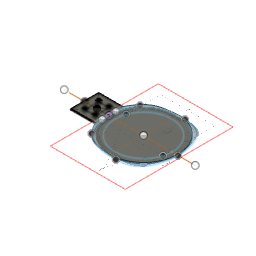
Support Joystick v4 (Autodesk Fusion 360 design; units mm, degrees)
Autodesk Fusion 360 part; units mm, degrees
sketch "Esquisse2" plane through (0, 0, 0) normal (0, 0, 1) x (1, 0, 0)
  line L0 (0, 0) -> (-70, 0)
  circle A0 centre (100, 0) radius 82.5
  line L1 (250, 0) -> (-130, 0)
  spline S0 degree 5 poles (0, 20) (0, 22.4882) (0.1779, 27.4114) (0.975, 34.6277) (3.4457, 44.3914) (10.1068, 57.8847) (21.3924, 73.1358) (35.9935, 85.4932) (52.8737, 92.6951) (72.095, 96.3693) (93.5882, 98.471) (117.0022, 100.5708) (140.5192, 100.2508) (161.4884, 92.9068) (178.6566, 78.1832) (191.1793, 56.7401) (197.2314, 35.6259) (199.4965, 18.2943) (200, 6.1899) (200, 0) knots 0 0 0 0 0 0 0.066667 0.133333 0.2 0.266667 0.333333 0.4 0.466667 0.533333 0.6 0.666667 0.733333 0.8 0.866667 0.933333 1 1 1 1 1 1
  line L2 (0, 0) -> (0, 40)
  line L3 (96.4605, 99.786) -> (143.5395, 100.214)
  line L4 (4.3857, 52.2523) -> (35.6143, 87.7477)
  spline S1 degree 5 poles (0, -20) (0, -22.4882) (0.1779, -27.4114) (0.975, -34.6277) (3.4457, -44.3914) (10.1068, -57.8847) (21.3924, -73.1358) (35.9935, -85.4932) (52.8737, -92.6951) (72.095, -96.3693) (93.5882, -98.471) (117.0022, -100.5708) (140.5192, -100.2508) (161.4884, -92.9068) (178.6566, -78.1832) (191.1793, -56.7401) (197.2314, -35.6259) (199.4965, -18.2943) (200, -6.1899) (200, 0) knots 0 0 0 0 0 0 0.066667 0.133333 0.2 0.266667 0.333333 0.4 0.466667 0.533333 0.6 0.666667 0.733333 0.8 0.866667 0.933333 1 1 1 1 1 1
  line L5 (200, 30) -> (200, -30)
  line L6 (0, 0) -> (0, -40)
  line L7 (4.3857, -52.2523) -> (35.6143, -87.7477)
  line L8 (96.4605, -99.786) -> (143.5395, -100.214)
  line L9 (200, -30) -> (200, 30)
  circle A1 centre (22.2756, 27.6617) radius 3.1
  circle A2 centre (179.3345, -22.6338) radius 3.1
  ellipse E0 centre (100, 0) end of major axis (100, 100) minor radius 100
  line L10 (100, -100) -> (100, 100)
  line L11 (200, 0) -> (0, 0)
  line L12 (-70, 40) -> (0, 40)
  line L13 (0, 40) -> (0, -40)
  line L14 (0, -40) -> (-70, -40)
  line L15 (-70, -40) -> (-70, 40)
  line L16 (-70, 40) -> (0, -40) construction
  line L17 (0, 40) -> (-70, -40) construction
  line L18 (0, -40) -> (10.9445, -57.8049)
  line L19 (0, 40) -> (10.9445, 57.8049)
  line L20 (-20, -20) -> (-50, -20)
  line L21 (-50, -20) -> (-50, 20)
  line L22 (-50, 20) -> (-20, 20)
  line L23 (-20, 20) -> (-20, -20)
  circle A3 centre (-50, 20) radius 4
  circle A4 centre (-20, 20) radius 4
  circle A5 centre (-50, -20) radius 4
  circle A6 centre (-20, -20) radius 4
  point P0 (-35, 0)
  point P1 (20, 70)
  point P2 (120, 100)
  point P3 (20, -70)
  point P4 (120, -100)
  point P5 (-35, 0)
  dimension "d3" = 70
  dimension "d5" = 165
  dimension "d6" = 6.2
  dimension "d7" = 6.2
  dimension "d18" = 70
  dimension "d19" = 80
  dimension "d28" = 20
  dimension "d29" = 8
  dimension "d32" = 30
  dimension "d33" = -40
  constraint coincident L0.start L2.start
  constraint horizontal L0
  constraint midpoint L0 P5
  constraint coincident L1 S0.end
  constraint midpoint S0.start L2
  constraint perpendicular L0 L2
  constraint midpoint P2 L3
  constraint midpoint P1 L4
  constraint midpoint S0.end L5
  constraint symmetric S0.start L1 S1.start
  constraint symmetric L1 P1 P3
  constraint symmetric L1 P2 P4
  constraint symmetric L1 L0.start L2.start
  constraint symmetric L1 L2.end L6.end
  constraint symmetric L1 L3.start L8.start
  constraint symmetric L1 L3.end L8.end
  constraint symmetric L1 L4.start L7.start
  constraint symmetric L1 L4.end L7.end
  constraint symmetric L1 L5.start L5.end
  constraint symmetric L1 L5.end L5.start
  constraint coincident A0 A1.centre
  constraint coincident A0 A2.centre
  constraint coincident E0 L10.start
  constraint coincident E0 L10.end
  constraint coincident S0.end E0
  constraint coincident L0.start E0
  constraint concentric A0 E0
  constraint perpendicular L1 L10
  constraint horizontal L12
  constraint perpendicular L12 L13
  constraint parallel L12 L14
  constraint parallel L13 L15
  constraint coincident L16 P5
  constraint coincident L17 P5
  constraint coincident P5 P0
  constraint coincident S1 L18.end
  constraint coincident L2.end L12.end
  constraint coincident S0 L19.end
  constraint coincident L21.end L22.start
  measures "d3" distance of L0.start L0.end
  measures "d5" diameter of A0
  measures "d6" diameter of A2
  measures "d7" diameter of A1
  measures "d18" distance of L6.end L14.end
  measures "d19" distance of L2.end L6.end
  measures "d29" diameter of A3
extrude "Extrusion1" add sketch "Esquisse2" along normal blind 3 contours L0 L1 L6 L13 L14 L15 L20 L21 L23 A5 A6 | A0 L1 S0 A1 E0 L10 L11 | L0 L1 L2 L12 L13 L15 L21 L22 L23 A3 A4 | A0 L1 S0 E0 L10 L11 | A0 L1 S1 E0 L10 L11 | L0 L1 L20 L21 L23 A5 A6 | L0 L1 L21 L22 L23 A3 A4 | A0 L1 L10 L11 | A0 L1 A1 L10 L11 | A0 L1 A2 L10 L11 | A0 L1 S1 A2 E0 L10 L11 | A0 L1 L10 L11
extrude "Extrusion2" cut sketch "Esquisse2" along normal blind 40 contours S1 E0 | S0 L3 E0 | S0 E0 | S1 L8 E0
extrude "Extrusion3" add sketch "Esquisse2" along normal blind 3 contours S1 L6 E0 L13 L18 | S0 L2 E0 L13 L19 | S0 L2 L13 L19 | S1 L6 L13 L18
